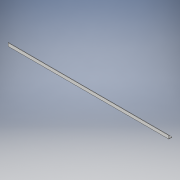
# Autodesk Inventor part: AluminumLchannel
Saved by Autodesk Inventor 2019 (Build 230136000, 136)
## iProperties
Created: 2019-01-21
Part Number: AluminumLchannel
Material: Generic
Document SubType Name: Modeling
Designer: josh
Density: 1 g/cm^3
Appearance: Default
Author: josh
Autodesk Inventor part; units mm, degrees
ref_plane "YZ Plane" through (0, 0, 0) normal (1, 0, 0) x (0, 1, 0)
ref_plane "XZ Plane" through (0, 0, 0) normal (0, 1, 0) x (-1, 0, 0)
ref_plane "XY Plane" through (0, 0, 0) normal (0, 0, 1) x (1, 0, 0)
sketch "Sketch1" plane through (0, 0, 0) normal (1, 0, 0) x (0, 1, 0)
  line L0 (0, 0) -> (0, -19.05)
  line L1 (0, 0) -> (19.05, 0)
  line L2 (19.05, -2.54) -> (2.54, -2.54)
  line L3 (2.54, -2.54) -> (2.54, -19.05)
  line L4 (2.54, -19.05) -> (0, -19.05)
  line L5 (19.05, 0) -> (19.05, -2.54)
  dimension "d0" = 19.05
  dimension "d2" = 19.05
  dimension "d3" = 2.54
  constraints: 12 end point, 2 horizontal, 1 perpendicular, 1 vertical, 1 other
  measures "d0" distance of L0.start L0.end
  measures "d2" distance of L0.start L1.end
  measures "d3" distance between parallel lines of L1 L2
extrude "Extrusion1" add sketch "Sketch1" against normal blind 990.6
body "Solid1"
